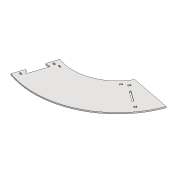
# Autodesk Inventor part: Level 1a - V2
Saved by Autodesk Inventor 2020 (Build 240168000, 168)
## iProperties
Created: 2020-07-30
Part Number: Level 1a - V2
Material: Generic
Document SubType Name: Modeling
Designer: Dan Wikman
Density: 1 g/cm^3
Appearance: Default
Author: Dan Wikman
Autodesk Inventor part; units mm, degrees
ref_plane "YZ Plane" through (0, 0, 0) normal (1, 0, 0) x (0, 1, 0)
ref_plane "XZ Plane" through (0, 0, 0) normal (0, 1, 0) x (-1, 0, 0)
ref_plane "XY Plane" through (0, 0, 0) normal (0, 0, 1) x (1, 0, 0)
sketch "Sketch1" plane through (0, 0, 0) normal (0, 1, 0) x (-1, 0, 0)
  line L0 (0, 0) -> (618.944217, 0)
  line L1 (0, 0) -> (191.264282, 588.650931)
  line L2 (0, 0) -> (-500.73639, 363.806283)
  line L3 (0, 0) -> (-500.73639, -363.806283)
  line L4 (0, 0) -> (191.264282, -588.650931)
  line L5 (396.643783, 3.75) -> (328.143783, 3.75)
  line L6 (328.143783, -3.75) -> (396.643783, -3.75)
  arc A0 (472.393783, 0) -> (145.977707, 449.273186) centre (0, 0) ccw
  arc A1 (77.993968, -240.040752) -> (252.393783, 0) centre (0, 0) ccw
  line L7 (289.893783, 3.75) -> (283.893782, 3.75)
  line L8 (283.893783, -3.75) -> (289.893781, -3.75)
  arc A2 (328.143783, 3.75) -> (326.393783, 2.000001) centre (328.143783, 2) ccw
  arc A3 (326.393783, -2) -> (328.143783, -3.75) centre (328.143783, -2) ccw
  line L9 (326.393783, 2.000001) -> (326.393783, -2)
  arc A4 (398.393783, 2) -> (396.643783, 3.75) centre (396.643783, 2) ccw
  arc A5 (396.643783, -3.75) -> (398.393783, -2.013555) centre (396.657285, -2.013555) ccw
  line L10 (398.393783, -2.013555) -> (398.393783, 2)
  line L11 (362.393783, -3.75) -> (362.393783, 32.980572)
  arc A6 (283.893782, 3.75) -> (282.143782, 2) centre (283.893782, 2) ccw
  arc A7 (282.143782, -2) -> (283.893783, -3.75) centre (283.893782, -2) ccw
  arc A8 (289.893781, -3.75) -> (291.64378, -2.000001) centre (289.89378, -2) ccw
  arc A9 (291.643783, 1.999999) -> (289.893783, 3.75) centre (289.893783, 2) ccw
  line L12 (291.643783, 1.999999) -> (291.64378, -2.000001)
  line L13 (282.143782, -2) -> (282.143782, 2)
  line L14 (434.893784, 3.75) -> (440.893785, 3.75)
  line L15 (440.893784, -3.75) -> (434.893785, -3.75)
  arc A10 (442.643785, 2) -> (440.893785, 3.75) centre (440.893785, 2) ccw
  arc A11 (440.893784, -3.75) -> (442.643785, -2) centre (440.893785, -2) ccw
  arc A12 (433.143787, -2.000001) -> (434.893785, -3.75) centre (434.893787, -2) ccw
  arc A13 (434.893784, 3.75) -> (433.143784, 1.999999) centre (434.893784, 2) ccw
  line L16 (433.143784, 1.999999) -> (433.143787, -2.000001)
  line L17 (442.643785, -2) -> (442.643785, 2)
  line L18 (131.946678, 412.562252) -> (135.750905, 411.326186)
  arc A14 (130.823108, 414.767381) -> (131.946678, 412.562252) centre (132.487457, 414.226601) ccw
  arc A15 (135.750905, 411.326186) -> (137.956032, 412.449755) centre (136.291684, 412.990536) ccw
  line L19 (139.810134, 418.156092) -> (137.956032, 412.449755)
  line L20 (130.823108, 414.767381) -> (132.67721, 420.473721)
  arc A16 (134.882339, 421.59729) -> (132.67721, 420.473721) centre (134.341559, 419.932941) ccw
  line L21 (138.686565, 420.361222) -> (134.882339, 421.59729)
  arc A17 (139.810134, 418.156092) -> (138.686565, 420.361222) centre (138.145785, 418.696873) ccw
  line L22 (125.025454, 378.272781) -> (121.208336, 379.513038)
  arc A18 (121.208336, 379.513038) -> (119.003208, 378.389469) centre (120.667557, 377.848689) ccw
  arc A19 (126.136132, 376.071841) -> (125.025454, 378.272781) centre (124.488846, 376.621273) ccw
  line L23 (119.003208, 378.389469) -> (97.835544, 313.242097)
  line L24 (98.959112, 311.036969) -> (102.763339, 309.800901)
  arc A20 (97.835544, 313.242097) -> (98.959112, 311.036969) centre (99.499893, 312.701317) ccw
  arc A21 (102.763339, 309.800901) -> (104.968468, 310.92447) centre (103.304119, 311.465249) ccw
  line L25 (104.968468, 310.92447) -> (126.136132, 376.071841)
  line L26 (88.220773, 277.987753) -> (92.024998, 276.751683)
  arc A22 (93.148567, 274.546556) -> (92.024998, 276.751683) centre (91.484217, 275.087334) ccw
  line L27 (91.294465, 268.840219) -> (93.148567, 274.546556)
  arc A23 (88.220773, 277.987753) -> (86.015643, 276.864185) centre (87.679992, 276.323405) ccw
  line L28 (86.015643, 276.864185) -> (84.161541, 271.157845)
  arc A24 (84.161541, 271.157845) -> (85.28511, 268.952716) centre (85.82589, 270.617065) ccw
  arc A25 (89.089336, 267.716648) -> (91.294465, 268.840219) centre (89.630116, 269.380997) ccw
  line L29 (89.089336, 267.716648) -> (85.28511, 268.952716)
  line L30 (-351.596252, 252.977495) -> (-349.245113, 256.213564)
  arc A26 (-354.040657, 252.590339) -> (-351.596252, 252.977495) centre (-353.012033, 254.006118) ccw
  arc A27 (-349.245113, 256.213564) -> (-349.632268, 258.657967) centre (-350.660894, 257.242188) ccw
  line L31 (-354.486369, 262.184678) -> (-349.632268, 258.657967)
  line L32 (-354.040657, 252.590339) -> (-358.89476, 256.117051)
  arc A28 (-359.281915, 258.561455) -> (-358.89476, 256.117051) centre (-357.866135, 257.532831) ccw
  line L33 (-356.930774, 261.797523) -> (-359.281915, 258.561455)
  arc A29 (-354.486369, 262.184678) -> (-356.930774, 261.797523) centre (-355.514994, 260.768898) ccw
  line L34 (-321.123804, 235.79899) -> (-323.482912, 232.551956)
  arc A30 (-323.482912, 232.551956) -> (-323.095756, 230.107553) centre (-322.067132, 231.523332) ccw
  arc A31 (-318.687367, 236.17518) -> (-321.123804, 235.79899) centre (-319.718947, 234.778302) ccw
  line L35 (-323.095756, 230.107553) -> (-267.678092, 189.844262)
  line L36 (-265.233688, 190.231418) -> (-262.882547, 193.467486)
  arc A32 (-267.678092, 189.844262) -> (-265.233688, 190.231418) centre (-266.649468, 191.260043) ccw
  arc A33 (-262.882547, 193.467486) -> (-263.269703, 195.91189) centre (-264.298327, 194.496111) ccw
  line L37 (-263.269703, 195.91189) -> (-318.687367, 236.17518)
  line L38 (-237.120346, 169.805881) -> (-234.769204, 173.041947)
  arc A34 (-232.324801, 173.429103) -> (-234.769204, 173.041947) centre (-233.353424, 172.013322) ccw
  line L39 (-227.4707, 169.902393) -> (-232.324801, 173.429103)
  arc A35 (-237.120346, 169.805881) -> (-236.733191, 167.361476) centre (-235.704567, 168.777256) ccw
  line L40 (-236.733191, 167.361476) -> (-231.879089, 163.834764)
  arc A36 (-231.879089, 163.834764) -> (-229.434685, 164.22192) centre (-230.850465, 165.250544) ccw
  arc A37 (-227.083544, 167.457988) -> (-227.4707, 169.902393) centre (-228.499324, 168.486612) ccw
  line L41 (-227.083544, 167.457988) -> (-229.434685, 164.22192)
  line L42 (-349.245113, -256.213562) -> (-351.596255, -252.977495)
  arc A38 (-349.632267, -258.657966) -> (-349.245113, -256.213562) centre (-350.660891, -257.242187) ccw
  arc A39 (-351.596255, -252.977495) -> (-354.040658, -252.59034) centre (-353.012035, -254.00612) ccw
  line L43 (-358.894758, -256.11705) -> (-354.040658, -252.59034)
  line L44 (-349.632267, -258.657966) -> (-354.48637, -262.184678)
  arc A40 (-356.930774, -261.797523) -> (-354.48637, -262.184678) centre (-355.514994, -260.768899) ccw
  line L45 (-359.281915, -258.561455) -> (-356.930774, -261.797523)
  arc A41 (-358.894758, -256.11705) -> (-359.281915, -258.561455) centre (-357.866135, -257.532831) ccw
  line L46 (-323.490879, -232.540991) -> (-321.131771, -235.788024)
  arc A42 (-321.131771, -235.788024) -> (-318.687367, -236.17518) centre (-319.715991, -234.7594) ccw
  arc A43 (-323.095756, -230.107553) -> (-323.490879, -232.540991) centre (-322.086023, -231.520303) ccw
  line L47 (-318.687367, -236.17518) -> (-263.269702, -195.91189)
  line L48 (-262.882547, -193.467487) -> (-265.233688, -190.231418)
  arc A44 (-263.269702, -195.91189) -> (-262.882547, -193.467487) centre (-264.298327, -194.496111) ccw
  arc A45 (-265.233688, -190.231418) -> (-267.678092, -189.844263) centre (-266.649468, -191.260043) ccw
  line L49 (-267.678092, -189.844263) -> (-323.095756, -230.107553)
  line L50 (-234.769207, -173.041947) -> (-237.120345, -169.805878)
  arc A46 (-236.73319, -167.361476) -> (-237.120345, -169.805878) centre (-235.704565, -168.777255) ccw
  line L51 (-231.87909, -163.834765) -> (-236.73319, -167.361476)
  arc A47 (-234.769207, -173.041947) -> (-232.324802, -173.429104) centre (-233.353426, -172.013324) ccw
  line L52 (-232.324802, -173.429104) -> (-227.470699, -169.902392)
  arc A48 (-227.470699, -169.902392) -> (-227.083544, -167.457988) centre (-228.499324, -168.486612) ccw
  arc A49 (-229.434685, -164.22192) -> (-231.87909, -163.834765) centre (-230.850465, -165.250544) ccw
  line L53 (-229.434685, -164.22192) -> (-227.083544, -167.457988)
  line L54 (135.750902, -411.326185) -> (131.946677, -412.562255)
  arc A50 (137.956032, -412.449754) -> (135.750902, -411.326185) centre (136.291683, -412.990533) ccw
  arc A51 (131.946677, -412.562255) -> (130.823108, -414.767382) centre (132.487458, -414.226604) ccw
  line L55 (132.67721, -420.47372) -> (130.823108, -414.767382)
  line L56 (137.956032, -412.449754) -> (139.810134, -418.156094)
  arc A52 (138.686565, -420.361222) -> (139.810134, -418.156094) centre (138.145785, -418.696873) ccw
  line L57 (134.882339, -421.59729) -> (138.686565, -420.361222)
  arc A53 (132.67721, -420.47372) -> (134.882339, -421.59729) centre (134.341559, -419.932941) ccw
  line L58 (121.195445, -379.517226) -> (125.012563, -378.27697)
  arc A54 (125.012563, -378.27697) -> (126.136132, -376.071841) centre (124.471783, -376.612621) ccw
  arc A55 (119.003208, -378.389469) -> (121.195445, -379.517226) centre (120.658838, -377.865719) ccw
  line L59 (126.136132, -376.071841) -> (104.968467, -310.924469)
  line L60 (102.76334, -309.8009) -> (98.959113, -311.036969)
  arc A56 (104.968467, -310.924469) -> (102.76334, -309.8009) centre (103.304119, -311.465249) ccw
  arc A57 (98.959113, -311.036969) -> (97.835544, -313.242097) centre (99.499893, -312.701317) ccw
  line L61 (97.835544, -313.242097) -> (119.003208, -378.389469)
  line L62 (92.024997, -276.751686) -> (88.220771, -277.987752)
  arc A58 (86.015643, -276.864184) -> (88.220771, -277.987752) centre (87.679992, -276.323402) ccw
  line L63 (84.161542, -271.157846) -> (86.015643, -276.864184)
  arc A59 (92.024997, -276.751686) -> (93.148567, -274.546557) centre (91.484219, -275.087337) ccw
  line L64 (93.148567, -274.546557) -> (91.294465, -268.840217)
  arc A60 (91.294465, -268.840217) -> (89.089337, -267.716648) centre (89.630116, -269.380997) ccw
  arc A61 (85.28511, -268.952716) -> (84.161542, -271.157846) centre (85.82589, -270.617065) ccw
  line L65 (85.28511, -268.952716) -> (89.089337, -267.716648)
  line L66 (-442.530326, 165.296089) -> (-220.837003, 122.203273)
  line L67 (-442.530326, -165.296089) -> (-220.837003, -122.203273)
  arc A62 (252.393783, 0) -> (-220.837003, 122.203273) centre (0, 0) ccw
  arc A63 (-220.837003, -122.203273) -> (77.993968, -240.040752) centre (0, 0) ccw
  arc A64 (145.977707, 449.273186) -> (-442.530326, 165.296089) centre (0, 0) ccw
  arc A65 (-442.530326, -165.296089) -> (472.393783, 0) centre (0, 0) ccw
  line L68 (115.678154, 400.516685) -> (82.986198, 299.90119)
  line L69 (84.650547, 297.61041) -> (108.748421, 297.61041)
  line L70 (110.41277, 295.31963) -> (90.955171, 235.435297)
  line L71 (138.866228, 382.890368) -> (158.992883, 444.833845)
  line L72 (118.634381, 401.156393) -> (135.910001, 382.25066)
  line L73 (123.116895, 378.892909) -> (127.272191, 391.703526) construction
  line L74 (100.861226, 310.418935) -> (96.699484, 297.61041) construction
  arc A66 (135.910001, 382.25066) -> (138.866228, 382.890368) centre (137.201879, 383.431148) ccw
  arc A67 (118.634381, 401.156393) -> (115.678154, 400.516685) centre (117.342503, 399.975905) ccw
  arc A68 (82.986198, 299.90119) -> (84.650547, 297.61041) centre (84.650547, 299.36041) ccw
  arc A69 (110.41277, 295.31963) -> (108.748421, 297.61041) centre (108.748421, 295.86041) ccw
  line L75 (407.062404, -13.75) -> (472.19363, -13.75)
  arc A70 (405.540481, -11.136142) -> (407.062404, -13.75) centre (407.062404, -12) ccw
  line L76 (418.182442, 11.136142) -> (405.540481, -11.136142)
  arc A71 (418.182442, 11.136142) -> (416.660519, 13.75) centre (416.660519, 12) ccw
  line L77 (416.660519, 13.75) -> (310.867126, 13.75)
  line L78 (309.202778, 11.45922) -> (316.64943, -11.45922)
  arc A72 (310.867126, 13.75) -> (309.202778, 11.45922) centre (310.867126, 12) ccw
  arc A73 (314.985081, -13.75) -> (316.64943, -11.45922) centre (314.985081, -12) ccw
  line L79 (314.985081, -13.75) -> (252.018966, -13.75)
  line L80 (112.712173, -391.388335) -> (132.838829, -453.331812)
  arc A74 (114.7278, -389.133174) -> (112.712173, -391.388335) centre (114.376522, -390.847556) ccw
  line L81 (139.816582, -394.273879) -> (114.7278, -389.133174)
  arc A75 (139.816582, -394.273879) -> (141.832208, -392.018718) centre (140.167859, -392.559497) ccw
  line L82 (141.832208, -392.018718) -> (109.140252, -291.403223)
  line L83 (106.447279, -290.528223) -> (86.951689, -304.692598)
  arc A76 (109.140252, -291.403223) -> (106.447279, -290.528223) centre (107.475903, -291.944002) ccw
  arc A77 (84.258716, -303.817598) -> (86.951689, -304.692598) centre (85.923065, -303.276818) ccw
  line L84 (84.258716, -303.817598) -> (64.801116, -243.933264)
  line L85 (277, 35.5) -> (273, 35.5)
  line L86 (271.25, 33.75) -> (271.25, 23.75)
  line L87 (273, 22) -> (277, 22)
  line L88 (278.75, 23.75) -> (278.75, 33.75)
  arc A78 (278.75, 33.75) -> (277, 35.5) centre (277, 33.75) ccw
  arc A79 (273, 35.5) -> (271.25, 33.75) centre (273, 33.75) ccw
  arc A80 (271.25, 23.75) -> (273, 22) centre (273, 23.75) ccw
  arc A81 (277, 22) -> (278.75, 23.75) centre (277, 23.75) ccw
  line L89 (277, -35.5) -> (273, -35.5)
  line L90 (271.25, -33.75) -> (271.25, -23.75)
  line L91 (273, -22) -> (277, -22)
  line L92 (278.75, -23.75) -> (278.75, -33.75)
  arc A82 (277, -35.5) -> (278.75, -33.75) centre (277, -33.75) ccw
  arc A83 (271.25, -33.75) -> (273, -35.5) centre (273, -33.75) ccw
  arc A84 (273, -22) -> (271.25, -23.75) centre (273, -23.75) ccw
  arc A85 (278.75, -23.75) -> (277, -22) centre (277, -23.75) ccw
  arc A86 (64.674464, 270.241029) -> (63.550895, 272.446158) centre (63.010115, 270.781809) ccw
  line L93 (63.550895, 272.446158) -> (54.04033, 275.536327)
  line L94 (63.438396, 266.436803) -> (64.674464, 270.241029)
  arc A87 (61.233267, 265.313234) -> (63.438396, 266.436803) centre (61.774047, 266.977583) ccw
  line L95 (51.835201, 274.412758) -> (50.599133, 270.608532)
  line L96 (51.722702, 268.403404) -> (61.233267, 265.313234)
  arc A88 (50.599133, 270.608532) -> (51.722702, 268.403404) centre (52.263482, 270.067753) ccw
  arc A89 (54.04033, 275.536327) -> (51.835201, 274.412758) centre (53.49955, 273.871979) ccw
  arc A90 (108.726079, 257.76785) -> (106.520951, 256.644281) centre (108.1853, 256.103501) ccw
  line L97 (105.284883, 252.840055) -> (106.520951, 256.644281)
  arc A91 (105.284883, 252.840055) -> (106.408452, 250.634926) centre (106.949232, 252.299275) ccw
  line L98 (108.726079, 257.76785) -> (118.236645, 254.67768)
  arc A92 (119.360214, 252.472552) -> (118.236645, 254.67768) centre (117.695865, 253.013331) ccw
  line L99 (115.919017, 247.544756) -> (106.408452, 250.634926)
  line L100 (119.360214, 252.472552) -> (118.124146, 248.668326)
  arc A93 (115.919017, 247.544756) -> (118.124146, 248.668326) centre (116.459797, 249.209105) ccw
  arc A94 (-211.553587, 183.059293) -> (-211.166432, 180.614889) centre (-210.137808, 182.030669) ccw
  line L101 (-207.930364, 178.263748) -> (-211.166432, 180.614889)
  arc A95 (-207.930364, 178.263748) -> (-205.48596, 178.650903) centre (-206.90174, 179.679527) ccw
  line L102 (-211.553587, 183.059293) -> (-205.675735, 191.149463)
  arc A96 (-203.231331, 191.536618) -> (-205.675735, 191.149463) centre (-204.259955, 190.120838) ccw
  line L103 (-199.608107, 186.741073) -> (-205.48596, 178.650903)
  line L104 (-203.231331, 191.536618) -> (-199.995263, 189.185477)
  arc A97 (-199.608107, 186.741073) -> (-199.995263, 189.185477) centre (-201.023887, 187.769697) ccw
  arc A98 (-211.166432, -180.614889) -> (-211.553587, -183.059293) centre (-210.137808, -182.030669) ccw
  line L105 (-211.553587, -183.059293) -> (-205.675735, -191.149463)
  line L106 (-207.930364, -178.263748) -> (-211.166432, -180.614889)
  arc A99 (-205.48596, -178.650903) -> (-207.930364, -178.263748) centre (-206.90174, -179.679527) ccw
  line L107 (-203.231331, -191.536618) -> (-199.995263, -189.185477)
  line L108 (-199.608107, -186.741073) -> (-205.48596, -178.650903)
  arc A100 (-199.995263, -189.185477) -> (-199.608107, -186.741073) centre (-201.023887, -187.769697) ccw
  arc A101 (-205.675735, -191.149463) -> (-203.231331, -191.536618) centre (-204.259955, -190.120838) ccw
  arc A102 (106.520951, -256.644281) -> (108.726079, -257.76785) centre (108.1853, -256.103501) ccw
  line L109 (108.726079, -257.76785) -> (118.236645, -254.67768)
  line L110 (105.284883, -252.840055) -> (106.520951, -256.644281)
  arc A103 (106.408452, -250.634926) -> (105.284883, -252.840055) centre (106.949232, -252.299275) ccw
  line L111 (119.360214, -252.472552) -> (118.124146, -248.668326)
  line L112 (115.919017, -247.544756) -> (106.408452, -250.634926)
  arc A104 (118.124146, -248.668326) -> (115.919017, -247.544756) centre (116.459797, -249.209105) ccw
  arc A105 (118.236645, -254.67768) -> (119.360214, -252.472552) centre (117.695865, -253.013331) ccw
  arc A106 (63.550895, -272.446158) -> (64.674464, -270.241029) centre (63.010115, -270.781809) ccw
  line L113 (63.438396, -266.436803) -> (64.674464, -270.241029)
  arc A107 (63.438396, -266.436803) -> (61.233267, -265.313234) centre (61.774047, -266.977583) ccw
  line L114 (63.550895, -272.446158) -> (54.04033, -275.536327)
  arc A108 (51.835201, -274.412758) -> (54.04033, -275.536327) centre (53.49955, -273.871979) ccw
  line L115 (51.722702, -268.403404) -> (61.233267, -265.313234)
  line L116 (51.835201, -274.412758) -> (50.599133, -270.608532)
  arc A109 (51.722702, -268.403404) -> (50.599133, -270.608532) centre (52.263482, -270.067753) ccw
  line L117 (-351.596252, 252.977495) -> (-355.245357, 247.912443)
  line L118 (-359.281915, 258.561455) -> (-362.91513, 253.454684)
  line L119 (-357.693865, 247.519615) -> (-362.517811, 251.024416)
  arc A110 (-362.91513, 253.454684) -> (-362.517811, 251.024416) centre (-361.489187, 252.440196) ccw
  arc A111 (-357.693865, 247.519615) -> (-355.245357, 247.912443) centre (-356.665241, 248.935394) ccw
  line L120 (-229.434685, 164.221921) -> (-233.08379, 159.156869)
  line L121 (-237.120347, 169.805881) -> (-240.753562, 164.69911)
  line L122 (-235.532298, 158.764041) -> (-240.356243, 162.268842)
  arc A112 (-240.753562, 164.69911) -> (-240.356243, 162.268842) centre (-239.327619, 163.684622) ccw
  arc A113 (-235.532298, 158.764041) -> (-233.08379, 159.156869) centre (-234.503673, 160.17982) ccw
  line L123 (-223.777058, -174.94374) -> (-228.601004, -178.448542)
  line L124 (-234.769206, -173.041949) -> (-231.035104, -178.07542)
  arc A114 (-231.035104, -178.07542) -> (-228.601004, -178.448542) centre (-229.629628, -177.032762) ccw
  arc A115 (-223.777058, -174.94374) -> (-223.394029, -172.49368) centre (-224.805682, -173.52796) ccw
  line L125 (-227.083545, -167.457988) -> (-223.394029, -172.49368)
  line L126 (97.23047, -266.885218) -> (99.073053, -272.556106)
  line L127 (92.024998, -276.751686) -> (97.966015, -274.755772)
  arc A116 (97.966015, -274.755772) -> (99.073053, -272.556106) centre (97.408704, -273.096886) ccw
  arc A117 (97.23047, -266.885218) -> (95.018687, -265.763826) centre (95.566121, -267.425998) ccw
  line L128 (89.089336, -267.716649) -> (95.018687, -265.763826)
  line L129 (283.868793, 9.999604) -> (289.831518, 9.999604)
  line L130 (291.643783, 2) -> (291.581431, 8.267014)
  arc A118 (291.581431, 8.267014) -> (289.831518, 9.999604) centre (289.831518, 8.249604) ccw
  arc A119 (283.868793, 9.999604) -> (282.118807, 8.242603) centre (283.868793, 8.249604) ccw
  line L131 (282.143783, 1.999999) -> (282.118807, 8.242603)
  line L132 (78.210093, 273.065313) -> (80.052676, 278.736201)
  line L133 (88.220772, 277.987754) -> (82.24122, 279.865068)
  arc A120 (82.24122, 279.865068) -> (80.052676, 278.736201) centre (81.717025, 278.195422) ccw
  arc A121 (78.210093, 273.065313) -> (79.340325, 270.858034) centre (79.874441, 272.524533) ccw
  line L134 (85.285111, 268.952717) -> (79.340325, 270.858034)
  line L135 (-356.930774, -261.797523) -> (-353.196672, -266.830994)
  arc A122 (-353.196672, -266.830994) -> (-350.762571, -267.204116) centre (-351.791195, -265.788336) ccw
  line L136 (-345.938626, -263.699314) -> (-350.762571, -267.204116)
  arc A123 (-345.938626, -263.699314) -> (-345.555597, -261.249254) centre (-346.96725, -262.283534) ccw
  line L137 (-349.245112, -256.213562) -> (-345.555597, -261.249254)
  line L138 (138.686565, -420.361222) -> (144.627582, -418.365308)
  arc A124 (144.627582, -418.365308) -> (145.73462, -416.165642) centre (144.070271, -416.706422) ccw
  line L139 (143.892037, -410.494753) -> (145.73462, -416.165642)
  arc A125 (143.892037, -410.494753) -> (141.680254, -409.373361) centre (142.227688, -411.035533) ccw
  line L140 (135.750903, -411.326185) -> (141.680254, -409.373361)
  line L141 (442.643785, 2) -> (442.581433, 8.267014)
  arc A126 (442.581433, 8.267014) -> (440.83152, 9.999604) centre (440.83152, 8.249604) ccw
  line L142 (434.868795, 9.999604) -> (440.83152, 9.999604)
  arc A127 (434.868795, 9.999604) -> (433.118809, 8.242603) centre (434.868795, 8.249604) ccw
  line L143 (433.143784, 1.999999) -> (433.118809, 8.242603)
  line L144 (134.882339, 421.59729) -> (128.902786, 423.474604)
  arc A128 (128.902786, 423.474604) -> (126.714243, 422.345737) centre (128.378591, 421.804957) ccw
  line L145 (124.871659, 416.674849) -> (126.714243, 422.345737)
  arc A129 (124.871659, 416.674849) -> (126.001891, 414.46757) centre (126.536008, 416.134069) ccw
  line L146 (131.946678, 412.562252) -> (126.001891, 414.46757)
  point P0 (115.5523, 343.498155)
  point P1 (-290.978535, 216.043535)
  point P2 (-295.386924, -209.975908)
  point P3 (108.419376, -345.815783)
  point P4 (137.937454, 380.031898)
  point P5 (97.940631, 311.906834)
  point P6 (104.098602, 309.905988)
  point P7 (119.873073, 379.40795)
  point P8 (404.05683, -13.75)
  point P9 (411.861461, 0)
  point P10 (312.926104, 0)
  point P11 (111.7834, -388.529865)
  point P12 (127.272191, -391.703526)
  point P13 (96.699484, -297.61041)
  point P14 (-363.919575, 252.042857)
  point P15 (-359.302101, 258.533082)
  point P16 (-352.164335, -268.222557)
  point P17 (146.270046, -417.813514)
  point P18 (442.564195, 9.999604)
  point P19 (127.249669, 423.993609)
  point P20 (85.285111, 268.952717)
  point P21 (88.18761, 277.998166)
  point P22 (-229.434685, 164.22192)
  point P23 (-237.140497, 169.777559)
  point P24 (131.946678, 412.562252)
  point P25 (134.849124, 421.607718)
  dimension "d4" = 360
  dimension "d6" = 7.5
  dimension "d7" = 7.5
  dimension "d9" = 68.5
  dimension "d10" = 7.5
  dimension "d11" = 7.5
  dimension "d12" = 3.5
  dimension "d13" = 3.5
  dimension "d19" = 360
  dimension "d21" = 25
  dimension "d25" = 10
  dimension "d26" = 10
  dimension "d27" = 1.75
  dimension "d30" = 144
  dimension "d32" = 271.25
  dimension "d33" = 7.5
  dimension "d34" = 13.5
  dimension "d36" = 1.75
  dimension "d40" = 20
  dimension "d46" = 0
  dimension "d47" = 8
  dimension "d48" = 1.75
  dimension "d67" = 1.75
  constraints: 294 end point, 265 point on circle, 130 centre point, 30 tangent, 26 point on line, 26 symmetric about line, 8 equal radius, 6 parallel, 5 horizontal, 5 midpoint, 2 coincident, 2 vertical, 1 equal length, 1 perpendicular, 390 other
  measures "d6" distance between parallel lines of L5 L6
  measures "d7" diameter of L6 L0
  measures "d9" distance of L6.start L6.end
  measures "d10" distance between parallel lines of L7 L8
  measures "d11" diameter of L7 L0
  measures "d12" diameter of A2
  measures "d13" diameter of A3
  measures "d21" angle of L35 L66
  measures "d25" distance between parallel lines of L23 L68
  measures "d26" distance between parallel lines of L25 L70
  measures "d27" radius of A66
  measures "d32" distance from line of point (0, 0) L86
  measures "d33" distance between parallel lines of L86 L88
  measures "d34" distance between parallel lines of L85 L87
  measures "d36" radius of A78
  measures "d40" distance from line of L5 A81.centre
  measures "d46" angle of L32 L119
  measures "d47" distance of L33.end point (-363.92, 252.043)
  measures "d48" radius of A110
  measures "d67" radius of A112
sketch "Sketch1 outline for Extrusion1" plane through (0, 0, 0) normal (0, 1, 0) x (-1, 0, 0)
  line L0 (108.748421, 297.61041) -> (84.650547, 297.61041)
  arc A0 (110.41277, 295.31963) -> (108.748421, 297.61041) centre (108.748421, 295.86041) ccw
  arc A1 (84.650547, 297.61041) -> (82.986198, 299.90119) centre (84.650547, 299.36041) cw
  line L1 (90.955171, 235.435297) -> (110.41277, 295.31963)
  line L2 (82.986198, 299.90119) -> (115.678154, 400.516685)
  arc A2 (-220.837003, 122.203273) -> (90.955171, 235.435297) centre (0, 0) cw
  arc A3 (115.678154, 400.516685) -> (118.634381, 401.156393) centre (117.342503, 399.975905) cw
  line L3 (-442.530326, 165.296089) -> (-220.837003, 122.203273)
  line L4 (118.634381, 401.156393) -> (135.910001, 382.25066)
  arc A4 (145.977707, 449.273186) -> (-442.530326, 165.296089) centre (0, 0) ccw
  arc A5 (135.910001, 382.25066) -> (138.866228, 382.890368) centre (137.201879, 383.431148) ccw
  arc A6 (158.992883, 444.833845) -> (145.977707, 449.273186) centre (0, 0) ccw
  line L5 (138.866228, 382.890368) -> (158.992883, 444.833845)
  line L6 (-262.882547, 193.467486) -> (-265.233688, 190.231418)
  arc A7 (-263.269703, 195.91189) -> (-262.882547, 193.467486) centre (-264.298327, 194.496111) cw
  line L7 (-318.687367, 236.17518) -> (-263.269703, 195.91189)
  arc A8 (-321.123804, 235.79899) -> (-318.687367, 236.17518) centre (-319.718947, 234.778302) cw
  line L8 (-323.482912, 232.551956) -> (-321.123804, 235.79899)
  arc A9 (-323.095756, 230.107553) -> (-323.482912, 232.551956) centre (-322.067132, 231.523332) cw
  line L9 (-267.678092, 189.844262) -> (-323.095756, 230.107553)
  arc A10 (-265.233688, 190.231418) -> (-267.678092, 189.844262) centre (-266.649468, 191.260043) cw
  line L10 (-237.120346, 169.805881) -> (-234.769204, 173.041947)
  arc A11 (-237.140497, 169.777559) -> (-237.120346, 169.805881) centre (-235.704567, 168.777256) cw
  line L11 (-240.753562, 164.69911) -> (-237.140497, 169.777559)
  arc A12 (-240.356243, 162.268842) -> (-240.753562, 164.69911) centre (-239.327619, 163.684622) cw
  line L12 (-235.532298, 158.764041) -> (-240.356243, 162.268842)
  arc A13 (-233.08379, 159.156869) -> (-235.532298, 158.764041) centre (-234.503673, 160.17982) cw
  line L13 (-229.434685, 164.22192) -> (-233.08379, 159.156869)
  line L14 (-227.083544, 167.457988) -> (-229.434685, 164.22192)
  arc A14 (-227.4707, 169.902393) -> (-227.083544, 167.457988) centre (-228.499324, 168.486612) cw
  line L15 (-232.324801, 173.429103) -> (-227.4707, 169.902393)
  arc A15 (-234.769204, 173.041947) -> (-232.324801, 173.429103) centre (-233.353424, 172.013322) cw
  line L16 (-207.930364, 178.263748) -> (-211.166432, 180.614889)
  arc A16 (-205.48596, 178.650903) -> (-207.930364, 178.263748) centre (-206.90174, 179.679527) cw
  line L17 (-199.608107, 186.741073) -> (-205.48596, 178.650903)
  arc A17 (-199.995263, 189.185477) -> (-199.608107, 186.741073) centre (-201.023887, 187.769697) cw
  line L18 (-203.231331, 191.536618) -> (-199.995263, 189.185477)
  arc A18 (-205.675735, 191.149463) -> (-203.231331, 191.536618) centre (-204.259955, 190.120838) cw
  line L19 (-211.553587, 183.059293) -> (-205.675735, 191.149463)
  arc A19 (-211.166432, 180.614889) -> (-211.553587, 183.059293) centre (-210.137808, 182.030669) cw
  line L20 (-359.281915, 258.561455) -> (-356.930774, 261.797523)
  arc A20 (-359.302101, 258.533082) -> (-359.281915, 258.561455) centre (-357.866135, 257.532831) cw
  line L21 (-362.91513, 253.454684) -> (-359.302101, 258.533082)
  arc A21 (-362.517811, 251.024416) -> (-362.91513, 253.454684) centre (-361.489187, 252.440196) cw
  line L22 (-357.693865, 247.519615) -> (-362.517811, 251.024416)
  arc A22 (-355.245357, 247.912443) -> (-357.693865, 247.519615) centre (-356.665241, 248.935394) cw
  line L23 (-351.596252, 252.977495) -> (-355.245357, 247.912443)
  line L24 (-349.245113, 256.213564) -> (-351.596252, 252.977495)
  arc A23 (-349.632268, 258.657967) -> (-349.245113, 256.213564) centre (-350.660894, 257.242188) cw
  line L25 (-354.486369, 262.184678) -> (-349.632268, 258.657967)
  arc A24 (-356.930774, 261.797523) -> (-354.486369, 262.184678) centre (-355.514994, 260.768898) cw
  line L26 (54.04033, 275.536327) -> (63.550895, 272.446158)
  arc A25 (51.835201, 274.412758) -> (54.04033, 275.536327) centre (53.49955, 273.871979) cw
  line L27 (50.599133, 270.608532) -> (51.835201, 274.412758)
  arc A26 (51.722702, 268.403404) -> (50.599133, 270.608532) centre (52.263482, 270.067753) cw
  line L28 (61.233267, 265.313234) -> (51.722702, 268.403404)
  arc A27 (63.438396, 266.436803) -> (61.233267, 265.313234) centre (61.774047, 266.977583) cw
  line L29 (64.674464, 270.241029) -> (63.438396, 266.436803)
  arc A28 (63.550895, 272.446158) -> (64.674464, 270.241029) centre (63.010115, 270.781809) cw
  line L30 (88.220773, 277.987753) -> (92.024998, 276.751683)
  arc A29 (88.18761, 277.998166) -> (88.220773, 277.987753) centre (87.679992, 276.323405) cw
  line L31 (82.24122, 279.865068) -> (88.18761, 277.998166)
  arc A30 (80.052676, 278.736201) -> (82.24122, 279.865068) centre (81.717025, 278.195422) cw
  line L32 (78.210093, 273.065313) -> (80.052676, 278.736201)
  arc A31 (79.340325, 270.858034) -> (78.210093, 273.065313) centre (79.874441, 272.524533) cw
  line L33 (85.285111, 268.952717) -> (79.340325, 270.858034)
  line L34 (89.089336, 267.716648) -> (85.285111, 268.952717)
  arc A32 (91.294465, 268.840219) -> (89.089336, 267.716648) centre (89.630116, 269.380997) cw
  line L35 (93.148567, 274.546556) -> (91.294465, 268.840219)
  arc A33 (92.024998, 276.751683) -> (93.148567, 274.546556) centre (91.484217, 275.087334) cw
  line L36 (134.882339, 421.59729) -> (138.686565, 420.361222)
  arc A34 (134.849124, 421.607718) -> (134.882339, 421.59729) centre (134.341559, 419.932941) cw
  line L37 (128.902786, 423.474604) -> (134.849124, 421.607718)
  arc A35 (126.714243, 422.345737) -> (128.902786, 423.474604) centre (128.378591, 421.804957) cw
  line L38 (124.871659, 416.674849) -> (126.714243, 422.345737)
  arc A36 (126.001891, 414.46757) -> (124.871659, 416.674849) centre (126.536008, 416.134069) cw
  line L39 (131.946678, 412.562252) -> (126.001891, 414.46757)
  line L40 (135.750905, 411.326186) -> (131.946678, 412.562252)
  arc A37 (137.956032, 412.449755) -> (135.750905, 411.326186) centre (136.291684, 412.990536) cw
  line L41 (139.810134, 418.156092) -> (137.956032, 412.449755)
  arc A38 (138.686565, 420.361222) -> (139.810134, 418.156092) centre (138.145785, 418.696873) cw
extrude "Extrusion1" add sketch "Sketch1 outline for Extrusion1" along normal blind 7
body "Solid1"
